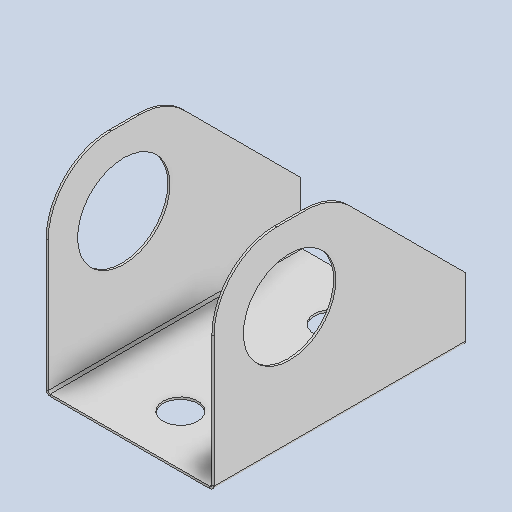
# Autodesk Inventor part: profile_mount-1
Saved by Autodesk Inventor 2025.2 (Build 292293000, 293)
## iProperties
Created: 2025-04-29
Part Number: profile_mount-1
Material: Generic
Document SubType Name: Sheet Metal
Designer: Caspe
Density: 1 g/cm^3
Sheet Metal Rule: Default_mm
Appearance: Default
Flat Pattern Width: 6 cm
Flat Pattern Length: 13.2262 cm
Flat Pattern Area: 79.3572 cm^2
Sheet Metal Width: 60,000 mm
Sheet Metal Length: 132,262 mm
Sheet Metal Area: 7935,717 mm^2
Author: Caspe
Autodesk Inventor part; units mm, degrees
ref_plane "YZ Plane" through (0, 0, 0) normal (1, 0, 0) x (0, 1, 0)
ref_plane "XZ Plane" through (0, 0, 0) normal (0, 1, 0) x (-1, 0, 0)
ref_plane "XY Plane" through (0, 0, 0) normal (0, 0, 1) x (1, 0, 0)
sketch "Sketch1" plane through (0, 0, 0) normal (0, 1, 0) x (-1, 0, 0)
  line L0 (0, 0) -> (40, 0)
  line L1 (40, 0) -> (40, -60)
  line L2 (40, -60) -> (0, -60)
  line L3 (0, -60) -> (0, 0)
  dimension "d0" = 40
  dimension "d1" = 60
  measures "d0" distance of L1.end L2.end
  measures "d1" distance of L0.end L1.end
extrude "Plate1" add sketch "Sketch1" along normal blind 0.5
sketch "Sketch2" plane through (-39.5, 0, 0) normal (-1, 0, 0) x (0, -1, 0)
  line L0 (0, -60) -> (0, 0)
  line L1 (0, 0) -> (-47, 0)
  line L2 (-47, 0) -> (-47, -60)
  line L3 (-47, -60) -> (0, -60)
  constraints: 6 end point, 1 horizontal, 1 perpendicular, 1 vertical
edge flange "Flange1" height 47 angle 90 thickness 0.5 bend radius 0.5 thickness toward (-1, 0, 0) relief straight relief width 0.5 relief depth 0.25 corner gap 0.5 corner form 0 edges at (-40, 0.5, -30) (0, 0.5, -30) wall of the first edge with corners at (-39.5, 0, -60) (-39.5, 0, 0) (-39.5, 47, 0) (-39.5, 47, -60)
bend "Bend1"
corner "Corner1"
sketch "Sketch4" plane through (-40, 47, -60) normal (-1, 0, 0) x (0, 0, 1)
  circle A0 centre (42, -18) radius 11
  line L0 (60, 0) -> (60, -46) projected
  line L1 (0, 0) -> (60, 0) projected
  point P0 (60, -47)
  dimension "d14" = 22
  dimension "d15" = 18
  dimension "d16" = 18
  constraints: 1 centre point
  measures "d14" diameter of A0
  measures "d15" distance from line of L0 A0.centre
  measures "d16" distance from line of L1 A0.centre
extrude "Cut1" cut sketch "Sketch4" against normal up to surface (40 mm away)
chamfer "Corner Chamfer1" distance 32 angle 45 2 edges at (-0.25, 47, -60) (-39.75, 47, -60)
fillet "Corner Round1" radius 15 4 edges at (-39.75, 47, -28) (-39.75, 47, 0) (-0.25, 47, 0) (-0.25, 47, -28)
sketch "Sketch5" plane through (0, 0.5, 0) normal (0, 1, 0) x (1, 0, 0)
  circle A0 centre (-20, 12) radius 4.15
  circle A1 centre (-20, 48) radius 4.15
  line L0 (-1, 0) -> (-39, 0) projected
  line L1 (-39, 60) -> (-1, 60) projected
  point P0 (0, 0)
  point P1 (-20, 0)
  dimension "d23" = 8.3
  dimension "d24" = 8.3
  dimension "d25" = 12
  dimension "d26" = 12
  constraints: 2 centre point, 1 midpoint
  measures "d23" diameter of A0
  measures "d24" diameter of A1
  measures "d25" distance of point (-20, 0) A0.centre
  measures "d26" distance from line of L1 A1.centre
extrude "Cut2" cut sketch "Sketch5" against normal up to surface (0.5 mm away)
equation "\"d17\" = Thickness"
equation "\"d27\" = Thickness"
equation "\"d2\" = Thickness"
equation "\"d3\" = BendReliefWidth"
equation "\"d4\" = BendReliefDepth"
equation "\"d5\" = MinimumRemnant"
equation "\"d6\" = TransitionRadius"
equation "\"d9\" = BendRadius"
equation "\"d10\" = CornerReliefSize"
equation "\"d11\" = GapSize"
equation "\"d12\" = JacobiRadiusSize"
equation "\"BendRadius\" = Thickness"
equation "\"BendReliefWidth\" = Thickness"
equation "\"BendReliefDepth\" = 0.5 * Thickness"
equation "\"CornerReliefSize\" = 4 * Thickness"
equation "\"MinimumRemnant\" = 2 * Thickness"
equation "\"TransitionRadius\" = BendRadius"
equation "\"JacobiRadiusSize\" = BendRadius"
equation "\"GapSize\" = Thickness"
equation "\"A_width\" = 46"
equation "\"A_joint_diameter\" = 16"
equation "\"A_B_spacing\" = 2"
equation "\"A_joint_tolerance\" = 3"
equation "\"l___________\" = 0"
equation "\"l__________\" = 0"
equation "\"l_________\" = 0"
equation "\"rivet_diameter\" = 3.35"
equation "\"plate_thickness\" = 3"
equation "\"l________\" = 0"
equation "\"L_Piston_Top\" = 25"
equation "\"L_Piston_Bottom\" = 21"
equation "\"Thickness\" = 0.5"
body "Solid1"
